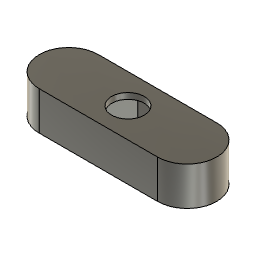
screw_holder_for_boat (Autodesk Fusion 360 design; units mm, degrees)
Autodesk Fusion 360 part; units mm, degrees
sketch "Sketch2" plane through (0, 0, 0) normal (0, 0, 1) x (1, 0, 0)
  line L0 (-4.5, 0) -> (4.5, 0)
  line L1 (-4.5, 0) -> (-2.25, 3.8971)
  line L2 (4.5, 0) -> (2.25, 3.8971)
  line L3 (4.5, 0) -> (9, 0) construction
  line L4 (-2.25, 3.8971) -> (2.25, 3.8971)
  line L5 (-4.5, 0) -> (-2.25, -3.8971)
  line L6 (4.5, 0) -> (2.25, -3.8971)
  line L7 (2.25, -3.8971) -> (-2.25, -3.8971)
  line L8 (-10, 5) -> (10, 5)
  line L9 (10, -5) -> (-10, -5)
  arc A0 (-10, 5) -> (-10, -5) centre (-10, 0) ccw
  arc A1 (10, -5) -> (10, 5) centre (10, 0) ccw
  circle A2 centre (0, 0) radius 2.75
  dimension "d15" = 120
  dimension "d16" = 120
  dimension "d17" = 5.5
  constraint horizontal L0
  constraint horizontal L3
  constraint parallel L2 L5
  constraint parallel L4 L7
  constraint tangent L8 A1
  constraint horizontal L8
  constraint tangent L9 A0
  constraint parallel L8 L9
  constraint coincident A2.centre origin
  measures "d15" angle of L0 L1
  measures "d16" angle of L2 L3
  measures "d17" diameter of A2
extrude "Extrude3" add sketch "Sketch2" along normal blind 6.5 contours L0 L1 L2 L4 A2 | L0 L5 L6 L7 A2 | L8 L9 A0 A1
extrude "Extrude4" cut sketch "Sketch2" along normal blind 5.5 contours L0 L1 L2 L4 A2 | L0 L5 L6 L7 A2
extrude "Extrude5" add sketch "Sketch2" along normal blind 1 contours L0 L1 L2 L4 A2 | L0 L5 L6 L7 A2
